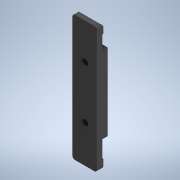
# Autodesk Inventor part: baseUBS2
Saved by Autodesk Inventor 2021.5 (Build 255421000, 421)
## iProperties
Created: 2025-06-30
Part Number: baseUBS2
Material: ABS NEGRO 4DLAB
Document SubType Name: Modeling
Designer: Joho_
Mass: 4.27796 g
Surface Area: 29.9551 cm^2
Volume: 4.78518 cm^3
Density: 0.894 g/cm^3
Appearance: Genérico
Author: Joho_
Autodesk Inventor part; units mm, degrees
ref_plane "YZ Plane" through (0, 0, 0) normal (1, 0, 0) x (0, 1, 0)
ref_plane "XZ Plane" through (0, 0, 0) normal (0, 1, 0) x (-1, 0, 0)
ref_plane "XY Plane" through (0, 0, 0) normal (0, 0, 1) x (1, 0, 0)
sketch "Boceto1" plane through (0, 0, 0) normal (0, 0, 1) x (1, 0, 0)
  circle A0 centre (0, 15) radius 2
  circle A1 centre (0, -15) radius 2
  line L0 (17.5, -36.1) -> (-17.5, -36.1)
  line L1 (-17.5, -36.1) -> (-17.5, 36.1)
  line L2 (-17.5, 36.1) -> (17.5, 36.1)
  line L3 (17.5, 36.1) -> (17.5, -36.1)
  line L4 (-17.5, 36.1) -> (17.5, 36.1)
  line L5 (17.5, 36.1) -> (17.5, 23.1)
  line L6 (17.5, 23.1) -> (-17.5, 23.1)
  line L7 (-17.5, 23.1) -> (-17.5, 36.1)
  line L8 (-17.5, 23.1) -> (17.5, 23.1)
  line L9 (17.5, 23.1) -> (17.5, 6.1)
  line L10 (17.5, 6.1) -> (-17.5, 6.1)
  line L11 (-17.5, 6.1) -> (-17.5, 23.1)
  line L12 (17.5, 6.1) -> (-17.5, 6.1)
  line L13 (-17.5, 6.1) -> (-17.5, -16.9)
  line L14 (-17.5, -16.9) -> (17.5, -16.9)
  line L15 (17.5, -16.9) -> (17.5, 6.1)
  line L16 (-17.5, 36.1) -> (17.5, 36.1)
  line L17 (17.5, 36.1) -> (17.5, 31.1)
  line L18 (17.5, 31.1) -> (-17.5, 31.1)
  line L19 (-17.5, 31.1) -> (-17.5, 36.1)
  line L20 (0, 36.1) -> (-7, 36.1)
  line L21 (0, 31.1) -> (-9.5, 31.1)
  line L22 (0, 23.1) -> (-9.75, 23.1)
  line L23 (-9.75, 23.1) -> (-9.5, 31.1)
  line L24 (0, 6.1) -> (-15, 6.1)
  line L25 (-15, 6.1) -> (-9.75, 23.1)
  line L26 (-17.5, -16.9) -> (17.5, -16.9)
  line L27 (17.5, -16.9) -> (17.5, -20.9)
  line L28 (17.5, -20.9) -> (-17.5, -20.9)
  line L29 (-17.5, -20.9) -> (-17.5, -16.9)
  line L30 (-15, 6.1) -> (-15, -16.9)
  line L31 (-15, -16.9) -> (-17.5, -20.9)
  arc A2 (-7, 36.1) -> (-9.5, 31.1) centre (-1.5455, 30.2478) ccw
  line L32 (7, -36) -> (-7, -36)
  line L33 (-7, -36) -> (-7, 36)
  line L34 (-7, 36) -> (7, 36)
  line L35 (7, 36) -> (7, -36)
  line L36 (7, -36) -> (-7, -36)
  line L37 (-7, -36) -> (-7, -31)
  line L38 (-7, -31) -> (7, -31)
  line L39 (7, -31) -> (7, -36)
  point P0 (0, 0)
  point P1 (-7, -20.9)
  point P2 (7, -20.9)
  point P3 (7, 23.1)
  point P4 (-7, 23.1)
  point P5 (7, -31)
  point P6 (-7, 31.1)
  point P7 (7, 31.1)
  dimension "d1" = 4
  dimension "d2" = 4
  dimension "d3" = 35
  dimension "d4" = 72.2
  dimension "d5" = 13
  dimension "d6" = 17
  dimension "d7" = 23
  dimension "d8" = 5
  dimension "d9" = 7
  dimension "d10" = 9.5
  dimension "d11" = 9.75
  dimension "d12" = 15
  dimension "d13" = 4
  dimension "d14" = 8
  dimension "d15" = 14
  dimension "d16" = 72
  dimension "d23" = 5
  constraints: 80 end point, 16 parallel, 11 point on line, 9 perpendicular, 8 horizontal, 4 midpoint, 3 centre point, 2 point on circle
  measures "d1" diameter of A0
  measures "d2" diameter of A1
  measures "d3" distance of L1.end L3.start
  measures "d4" distance of L1.start L1.end
  measures "d5" distance of L5.start L6.start
  measures "d6" distance of L9.start L15.end
  measures "d7" distance of L13.end L12.end
  measures "d8" distance of L17.start L18.start
  measures "d9" distance of L20.start L20.end
  measures "d10" distance of L21.start L21.end
  measures "d11" distance of L22.start L25.end
  measures "d12" distance of L24.start L25.start
  measures "d13" distance of L26.end L27.end
  measures "d14" radius of A2
  measures "d15" distance of L33.end L34.end
  measures "d16" distance of L32.end L33.end
  measures "d23" distance of L36.end L37.end
extrude "base" add sketch "Boceto1" along normal blind 3 contours A1 L14 L33 L10 L35 | A1 L14 L35 L28 L33 | L28 L35 L38 L33 | L33 L6 L35 L10 | L38 L35 L32 L33 | L33 L18 L35 L6 | L33 L34 L35 L18
extrude "base2" add sketch "Boceto1" against normal blind 3 contours A1 L14 L33 L10 L35 | A1 L14 L35 L28 L33 | L33 L6 L35 L10
extrude "Extrusión3" add sketch "Boceto1" against normal blind 0.6 contours L38 L35 L32 L33 | L33 L34 L35 L18
fillet "Empalme2" radius 1.5 6 edges at (0, 36, -0.6) (0, -36, -0.6) (7, -36, 1.2) (7, 36, 1.2) (-7, 36, 1.2) (-7, -36, 1.2)
